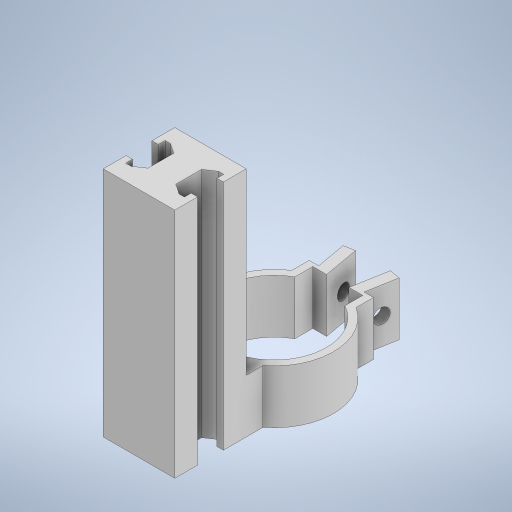
# Autodesk Inventor part: USB_camera
Saved by Autodesk Inventor 2024.3 (Build 283343000, 343)
## iProperties
Created: 2025-10-23
Part Number: USB_camera
Material: 일반
Document SubType Name: Modeling
Designer: joung
Density: 1 g/cm^3
Appearance: 기본값
Author: joung
Autodesk Inventor part; units mm, degrees
ref_plane "YZ Plane" through (0, 0, 0) normal (1, 0, 0) x (0, 1, 0)
ref_plane "XZ Plane" through (0, 0, 0) normal (0, 1, 0) x (-1, 0, 0)
ref_plane "XY Plane" through (0, 0, 0) normal (0, 0, 1) x (1, 0, 0)
sketch "스케치1" plane through (0, 0, 0) normal (0, 1, 0) x (-1, 0, 0)
  arc A0 (0, -14.55) -> (-2.5266, -14.329) centre (0, 0) ccw
  line L0 (-2.5656, -14.55) -> (-7, -14.55)
  line L1 (7, -14.55) -> (7, -12.7555)
  line L2 (-7, -14.55) -> (-7, -12.7555)
  arc A1 (2.8739, -16.2986) -> (-2.8739, -16.2986) centre (0, 0) ccw
  line L3 (7, -12.7555) -> (7, -17.7555)
  line L4 (-7, -12.7555) -> (-7, -17.7555)
  line L5 (-7, -17.7555) -> (-9, -17.7555)
  line L6 (-9, -17.7555) -> (-9, -13.8889)
  line L7 (7, -17.7555) -> (9, -17.7555)
  line L8 (9, -17.7555) -> (9, -13.8889)
  line L9 (0, 0) -> (23.7529, 0) construction
  line L10 (0, 0) -> (23.7529, 0) construction
  line L11 (4.1247, -23.3921) -> (7.0791, -22.8711)
  line L12 (7.0791, -22.8711) -> (6.1771, -17.7555)
  line L13 (-4.1247, -23.3921) -> (-7.0791, -22.8711)
  line L14 (-7.0791, -22.8711) -> (-6.1771, -17.7555)
  line L15 (-7, -17.7555) -> (-3.1308, -17.7555)
  line L16 (-9, -17.7555) -> (-9, -18.7555)
  line L17 (-9, -18.7555) -> (-6.3534, -18.7555)
  line L18 (9, -17.7555) -> (9, -18.7555)
  line L19 (9, -18.7555) -> (6.3534, -18.7555)
  line L20 (7, -17.7555) -> (6.1771, -17.7555)
  line L21 (6.1771, -17.7555) -> (3.1308, -17.7555)
  line L22 (0, 0) -> (-2.8739, -16.2986)
  line L23 (-3.1308, -17.7555) -> (-4.1247, -23.3921)
  line L24 (0, 0) -> (2.8739, -16.2986)
  line L25 (3.1308, -17.7555) -> (4.1247, -23.3921)
  line L26 (-7, -14.55) -> (-2.5656, -14.55)
  line L27 (0, -14.55) -> (7, -14.55)
  line L28 (3.1308, -17.7555) -> (4.8673, -27.6036)
  line L29 (4.8673, -27.6036) -> (7.8217, -27.0826)
  line L30 (7.8217, -27.0826) -> (7.0791, -22.8711)
  line L31 (-3.1308, -17.7555) -> (-4.8673, -27.6036)
  line L32 (-4.8673, -27.6036) -> (-7.8217, -27.0826)
  line L33 (-7.8217, -27.0826) -> (-7.0791, -22.8711)
  point P0 (-7, -14.9967)
  dimension "d0" = 29.1
  dimension "d1" = 7
  dimension "d2" = 14
  dimension "d3" = 2
  dimension "d4" = 5
  dimension "d5" = 2
  dimension "d6" = 2
  dimension "d7" = 5
  dimension "d10" = 3
  dimension "d11" = 1
  dimension "d14" = 10
  dimension "d15" = 10
  constraints: 68 end point, 12 perpendicular, 10 point on line, 8 point on circle, 5 horizontal, 3 vertical, 2 centre point, 1 coincident, 1 parallel, 1 tangent
  measures "d0" diameter of A0
  measures "d1" distance of L27.start L0.end
  measures "d2" distance of L0.end L1.start
  measures "d3" radial gap between concentric circles of A0 A1
  measures "d4" distance of L1.end L3.end
  measures "d5" distance of L4.end L5.end
  measures "d6" distance of L3.end L7.end
  measures "d7" distance of L2.end L4.end
  measures "d10" distance of L11.start L11.end
  measures "d11" distance of L5.end L16.end
  measures "d14" distance of L21.end L28.end
  measures "d15" distance of L15.end L31.end
extrude "돌출1" add sketch "스케치1" along normal blind 15 contours A0 L2 L4 A1 L3 L1 | A1 L8 L7 L3 | L4 L5 L6 A1 | L7 L18 L19 L12 L20 | L15 L14 L17 L16 L5 | L12 L11 L25 L21 | L15 L23 L13 L14 | L30 L29 L28 L11 | L13 L31 L32 L33
sketch "스케치2" plane through (7.8217, 0, -27.0826) normal (0.9848, 0, 0.1736) x (0.1736, 0, -0.9848)
  line L0 (0, 0) -> (0, 15) projected
  line L1 (-8.4556, 0) -> (-8.4556, 15) projected
  line L2 (0, 15) -> (-8.4556, 15)
  circle A0 centre (-4.2278, 7.5) radius 2.1
  point P0 (-28.0294, 0)
  dimension "d16" = 4.2
  constraints: 2 end point, 1 centre point, 1 perpendicular
  measures "d16" diameter of A0
extrude "돌출2" cut sketch "스케치2" against normal up to surface (3 mm away)
sketch "스케치3" plane through (-6.3534, 0, -18.7555) normal (-0.9848, 0, 0.1736) x (0.1736, 0, 0.9848)
  line L0 (1.5444, 0) -> (-8.4556, 0) projected
  line L1 (0, 0) -> (0, 15) projected
  line L2 (-8.4556, 0) -> (0, 0)
  circle A0 centre (-4.2278, 7.5) radius 2.1
  point P0 (19.5738, 0)
  dimension "d19" = 4.2
  constraints: 2 end point, 1 centre point, 1 perpendicular
  measures "d19" diameter of A0
extrude "돌출3" cut sketch "스케치3" against normal up to surface (3 mm away)
sketch "스케치4" plane through (0, 15, 0) normal (0, 1, 0) x (1, 0, 0)
  circle A0 centre (0, 0) radius 16.55
  line L0 (-10, -22.55) -> (10, -22.55)
  line L1 (10, -22.55) -> (10, -10.55)
  line L2 (10, -10.55) -> (-10, -10.55)
  line L3 (-10, -10.55) -> (-10, -22.55)
  arc A1 (-9, 13.8889) -> (9, 13.8889) centre (0, 0) ccw projected
  line L4 (-10, -22.55) -> (10, -10.55) construction
  line L5 (10, -22.55) -> (-10, -10.55) construction
  point P0 (0, -16.55)
  point P1 (10, -13.1872)
  point P2 (-10, -13.1872)
  dimension "d22" = 20
  dimension "d23" = 12
  constraints: 12 end point, 2 midpoint, 2 parallel, 1 centre point, 1 coincident, 1 horizontal, 1 perpendicular, 1 point on circle
  measures "d22" distance of L2.end L1.end
  measures "d23" distance of L1.end L0.end
extrude "돌출4" add sketch "스케치4" against normal up to surface (15 mm away) contours L1 L0 L3 A0
sketch "스케치5" plane through (0, 15, 0) normal (0, 1, 0) x (1, 0, 0)
  line L0 (-10, -13.1872) -> (-10, -22.55) projected
  line L1 (-10, -17.8686) -> (10, -17.8686)
  line L2 (10, -17.8686) -> (10, -37.8686)
  line L3 (10, -37.8686) -> (-10, -37.8686)
  line L4 (-10, -37.8686) -> (-10, -17.8686)
  point P0 (0, 0)
  dimension "d26" = 20
  dimension "d27" = 20
  constraints: 8 end point, 2 parallel, 1 horizontal, 1 midpoint, 1 perpendicular
  measures "d26" distance of L2.end L3.end
  measures "d27" distance of L1.end L2.end
extrude "돌출5" add sketch "스케치5" along normal blind 50 and the other way blind 15
sketch "스케치6" plane through (0, 65, 0) normal (0, 1, 0) x (1, 0, 0)
  line L0 (-10, -13.1872) -> (-10, -17.8686) projected
  line L1 (-10, -37.8686) -> (-10, -13.1872) projected
  line L2 (-10, -17.8686) -> (-10, -37.8686)
  line L3 (-10, -37.8686) -> (-10, -27.8686)
  line L4 (-10, -27.8686) -> (-10, -24.7686)
  line L5 (-10, -27.8686) -> (-10, -24.2686)
  line L6 (-10, -27.8686) -> (-10, -22.3686)
  line L7 (-10, -24.2686) -> (-8.2, -24.2686)
  line L8 (-8.2, -24.2686) -> (-8.2, -22.3686)
  line L9 (-8.2, -22.3686) -> (-6.7, -22.3686)
  line L10 (-10, -22.3686) -> (-3.9, -22.3686)
  line L11 (-6.7, -22.3686) -> (-3.9, -24.2686)
  line L12 (-3.9, -24.2686) -> (-3.9, -27.8686)
  line L13 (-10, -27.8686) -> (-3.9, -27.8686)
  line L14 (-10, -31.4686) -> (-8.2, -31.4686)
  line L15 (-8.2, -31.4686) -> (-8.2, -33.3686)
  line L16 (-8.2, -33.3686) -> (-6.7, -33.3686)
  line L17 (-6.7, -33.3686) -> (-3.9, -31.4686)
  line L18 (-3.9, -31.4686) -> (-3.9, -27.8686)
  line L19 (-10, -27.8686) -> (-10, -17.8686)
  point P0 (0, 0)
  point P1 (-10, -31.4686)
  dimension "d32" = 3.1
  dimension "d33" = 3.6
  dimension "d34" = 5.5
  dimension "d35" = 1.8
  dimension "d36" = 1.5
  dimension "d37" = 6.1
  dimension "d40" = 10
  constraints: 36 end point, 5 symmetric about line, 4 point on line, 3 perpendicular, 2 collinear, 2 horizontal, 1 midpoint, 1 vertical
  measures "d32" distance of L3.end L4.end
  measures "d33" distance of L3.end L5.end
  measures "d34" distance of L3.end L6.end
  measures "d35" distance of L5.end L7.end
  measures "d36" distance of L8.end L9.end
  measures "d37" distance of L6.end L10.end
  measures "d40" distance of L13.start L0.end
extrude "돌출6" cut sketch "스케치6" against normal through all contours L1 L13 L18 L17 L16 L15 L14 | L1 L7 L8 L9 L11 L12 L13
mirror "미러1" about plane through (0, 0, 0) normal (1, 0, 0) of "돌출6"
